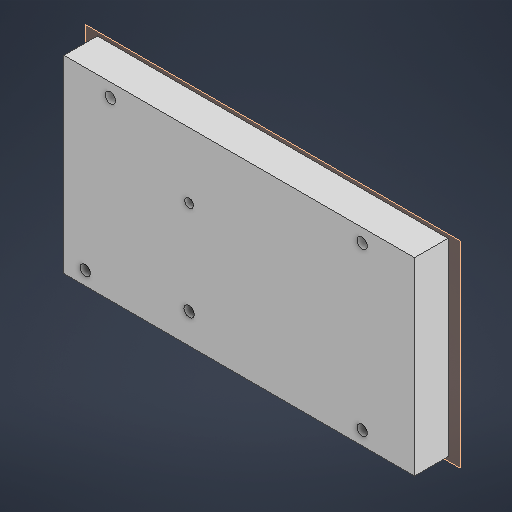
# Autodesk Inventor part: SAFRS-P-0040
Saved by Autodesk Inventor 2026.2 (Build 302298000, 298)
## iProperties
Created: 2025-11-26
Part Number: SAFRS-P-0040
Material: 일반
Document SubType Name: Modeling
Designer: jaewook
Density: 1 g/cm^3
Appearance: 기본값
Author: jaewook
Title: Mega Base
Autodesk Inventor part; units mm, degrees
ref_plane "YZ Plane" through (0, 0, 0) normal (1, 0, 0) x (0, 1, 0)
ref_plane "XZ Plane" through (0, 0, 0) normal (0, 1, 0) x (-1, 0, 0)
ref_plane "XY Plane" through (0, 0, 0) normal (0, 0, 1) x (1, 0, 0)
ref_plane "작업 평면1" through (0, 0, 0) normal (0, 0, 1) x (1, 0, 0)
sketch "스케치1" plane through (0, 0, 0) normal (0, 0, 1) x (1, 0, 0)
  line L0 (-103.1, 54.9162) -> (1.5, 54.9162)
  line L1 (1.5, 54.9162) -> (1.5, -1.5)
  line L2 (1.5, -1.5) -> (-103.1, -1.5)
  line L3 (-103.1, -1.5) -> (-103.1, 54.9162)
  line L4 (0, 1.524) -> (0, 51.8922) projected
  line L5 (-99.06, 40.7162) -> (-101.6, 38.1762) projected
  line L6 (-101.6, 38.1762) -> (-101.6, 3.556) projected
  line L7 (-101.6, 3.556) -> (-98.044, 0) projected
  line L8 (-98.044, 0) -> (-1.524, 0) projected
  line L9 (-1.524, 0) -> (0, 1.524) projected
  line L10 (0, 1.524) -> (0, 51.8922) projected
  line L11 (0, 51.8922) -> (-1.524, 53.4162) projected
  line L12 (-1.524, 53.4162) -> (-97.2966, 53.4162) projected
  line L13 (-97.2966, 53.4162) -> (-99.06, 51.6528) projected
  line L14 (-99.06, 51.6528) -> (-99.06, 40.7162) projected
  circle A0 centre (-89.2556, 50.8762) radius 1.5621 projected
  circle A1 centre (-65.7479, 35.4347) radius 1.3153 projected
  circle A2 centre (-65.7479, 7.4185) radius 1.5621 projected
  circle A3 centre (-96.7486, 2.54) radius 1.5621 projected
  circle A4 centre (-14.1224, 2.54) radius 1.5621 projected
  circle A5 centre (-14.1224, 50.8762) radius 1.5621 projected
  line L15 (-91.7703, 3.1886) -> (-92.8414, 3.1886) projected
  line L16 (-91.7703, 1.1751) -> (-91.7703, 3.1886) projected
  line L17 (-92.8414, 1.1751) -> (-91.7703, 1.1751) projected
  line L18 (-92.8414, 3.1886) -> (-92.8414, 1.1751) projected
  line L19 (-86.6903, 1.1751) -> (-86.6903, 3.1886) projected
  line L20 (-87.7614, 1.1751) -> (-86.6903, 1.1751) projected
  line L21 (-87.7614, 3.1886) -> (-87.7614, 1.1751) projected
  line L22 (-86.6903, 3.1886) -> (-87.7614, 3.1886) projected
  line L23 (-81.6103, 1.1751) -> (-81.6103, 3.1886) projected
  line L24 (-82.6814, 1.1751) -> (-81.6103, 1.1751) projected
  line L25 (-82.6814, 3.1886) -> (-82.6814, 1.1751) projected
  line L26 (-81.6103, 3.1886) -> (-82.6814, 3.1886) projected
  line L27 (-76.5303, 1.1751) -> (-76.5303, 3.1886) projected
  line L28 (-77.6014, 1.1751) -> (-76.5303, 1.1751) projected
  line L29 (-77.6014, 3.1886) -> (-77.6014, 1.1751) projected
  line L30 (-76.5303, 3.1886) -> (-77.6014, 3.1886) projected
  line L31 (-68.6825, 3.4297) -> (-69.7244, 3.4297) projected
  line L32 (-68.6825, 1.346) -> (-68.6825, 3.4297) projected
  line L33 (-69.7244, 1.346) -> (-68.6825, 1.346) projected
  line L34 (-69.7244, 3.4297) -> (-69.7244, 1.346) projected
  line L35 (-63.6025, 1.346) -> (-63.6025, 3.4297) projected
  line L36 (-64.6444, 1.346) -> (-63.6025, 1.346) projected
  line L37 (-64.6444, 3.4297) -> (-64.6444, 1.346) projected
  line L38 (-63.6025, 3.4297) -> (-64.6444, 3.4297) projected
  line L39 (-58.5225, 1.346) -> (-58.5225, 3.4297) projected
  line L40 (-59.5644, 1.346) -> (-58.5225, 1.346) projected
  line L41 (-59.5644, 3.4297) -> (-59.5644, 1.346) projected
  line L42 (-58.5225, 3.4297) -> (-59.5644, 3.4297) projected
  line L43 (-53.4425, 1.346) -> (-53.4425, 3.4297) projected
  line L44 (-54.4844, 1.346) -> (-53.4425, 1.346) projected
  line L45 (-54.4844, 3.4297) -> (-54.4844, 1.346) projected
  line L46 (-53.4425, 3.4297) -> (-54.4844, 3.4297) projected
  line L47 (-45.4737, 3.6867) -> (-46.5774, 3.6867) projected
  line L48 (-45.4737, 1.6118) -> (-45.4737, 3.6867) projected
  line L49 (-46.5774, 1.6118) -> (-45.4737, 1.6118) projected
  line L50 (-46.5774, 3.6867) -> (-46.5774, 1.6118) projected
  line L51 (-40.3937, 1.6118) -> (-40.3937, 3.6867) projected
  line L52 (-41.4974, 1.6118) -> (-40.3937, 1.6118) projected
  line L53 (-41.4974, 3.6867) -> (-41.4974, 1.6118) projected
  line L54 (-40.3937, 3.6867) -> (-41.4974, 3.6867) projected
  line L55 (-35.3137, 1.6118) -> (-35.3137, 3.6867) projected
  line L56 (-36.4174, 1.6118) -> (-35.3137, 1.6118) projected
  line L57 (-36.4174, 3.6867) -> (-36.4174, 1.6118) projected
  line L58 (-35.3137, 3.6867) -> (-36.4174, 3.6867) projected
  circle A6 centre (-97.5648, 7.2848) radius 0.5739 projected
  circle A7 centre (-95.0248, 7.2848) radius 0.5739 projected
  circle A8 centre (-95.0248, 9.8248) radius 0.5739 projected
  circle A9 centre (-95.0248, 12.3648) radius 0.5739 projected
  circle A10 centre (-95.0248, 14.9048) radius 0.5739 projected
  circle A11 centre (-95.0248, 17.4448) radius 0.5739 projected
  circle A12 centre (-95.0248, 19.9848) radius 0.5739 projected
  circle A13 centre (-95.0248, 22.5248) radius 0.5739 projected
  circle A14 centre (-95.0248, 25.0648) radius 0.5739 projected
  circle A15 centre (-95.0248, 27.6048) radius 0.5739 projected
  circle A16 centre (-95.0248, 30.1448) radius 0.5739 projected
  circle A17 centre (-95.0248, 32.6848) radius 0.5739 projected
  circle A18 centre (-95.0248, 35.2248) radius 0.5739 projected
  circle A19 centre (-95.0248, 37.7648) radius 0.5739 projected
  circle A20 centre (-95.0248, 40.3048) radius 0.5739 projected
  circle A21 centre (-95.0248, 42.8448) radius 0.5739 projected
  circle A22 centre (-95.0248, 45.3848) radius 0.5739 projected
  circle A23 centre (-95.0248, 47.9248) radius 0.5739 projected
  circle A24 centre (-95.0248, 50.4648) radius 0.5739 projected
  line L59 (-81.8933, 50.0717) -> (-81.8933, 51.6679) projected
  line L60 (-82.3984, 50.0717) -> (-81.8933, 50.0717) projected
  line L61 (-82.3984, 51.6679) -> (-82.3984, 50.0717) projected
  line L62 (-81.8933, 51.6679) -> (-82.3984, 51.6679) projected
  line L63 (-76.8133, 50.0717) -> (-76.8133, 51.6679) projected
  line L64 (-77.3184, 50.0717) -> (-76.8133, 50.0717) projected
  line L65 (-77.3184, 51.6679) -> (-77.3184, 50.0717) projected
  line L66 (-76.8133, 51.6679) -> (-77.3184, 51.6679) projected
  line L67 (-71.7333, 50.0717) -> (-71.7333, 51.6679) projected
  line L68 (-72.2384, 50.0717) -> (-71.7333, 50.0717) projected
  line L69 (-72.2384, 51.6679) -> (-72.2384, 50.0717) projected
  line L70 (-71.7333, 51.6679) -> (-72.2384, 51.6679) projected
  line L71 (-63.4227, 51.9137) -> (-64.2563, 51.9137) projected
  line L72 (-63.4227, 50.0717) -> (-63.4227, 51.9137) projected
  line L73 (-64.2563, 50.0717) -> (-63.4227, 50.0717) projected
  line L74 (-64.2563, 51.9137) -> (-64.2563, 50.0717) projected
  line L75 (-58.3427, 50.0717) -> (-58.3427, 51.9137) projected
  line L76 (-59.1763, 50.0717) -> (-58.3427, 50.0717) projected
  line L77 (-59.1763, 51.9137) -> (-59.1763, 50.0717) projected
  line L78 (-58.3427, 51.9137) -> (-59.1763, 51.9137) projected
  line L79 (-53.2627, 50.0717) -> (-53.2627, 51.9137) projected
  line L80 (-54.0963, 50.0717) -> (-53.2627, 50.0717) projected
  line L81 (-54.0963, 51.9137) -> (-54.0963, 50.0717) projected
  line L82 (-53.2627, 51.9137) -> (-54.0963, 51.9137) projected
  line L83 (-48.1827, 50.0717) -> (-48.1827, 51.9137) projected
  line L84 (-49.0163, 50.0717) -> (-48.1827, 50.0717) projected
  line L85 (-49.0163, 51.9137) -> (-49.0163, 50.0717) projected
  line L86 (-48.1827, 51.9137) -> (-49.0163, 51.9137) projected
  line L87 (-41.4974, 51.9137) -> (-42.4723, 51.9137) projected
  line L88 (-41.4974, 50.0717) -> (-41.4974, 51.9137) projected
  line L89 (-42.4723, 50.0717) -> (-41.4974, 50.0717) projected
  line L90 (-42.4723, 51.9137) -> (-42.4723, 50.0717) projected
  line L91 (-36.4174, 50.0717) -> (-36.4174, 51.9137) projected
  line L92 (-37.3923, 50.0717) -> (-36.4174, 50.0717) projected
  line L93 (-37.3923, 51.9137) -> (-37.3923, 50.0717) projected
  line L94 (-36.4174, 51.9137) -> (-37.3923, 51.9137) projected
  line L95 (-31.3374, 50.0717) -> (-31.3374, 51.9137) projected
  line L96 (-32.3123, 50.0717) -> (-31.3374, 50.0717) projected
  line L97 (-32.3123, 51.9137) -> (-32.3123, 50.0717) projected
  line L98 (-31.3374, 51.9137) -> (-32.3123, 51.9137) projected
  line L99 (-26.2574, 50.0717) -> (-26.2574, 51.9137) projected
  line L100 (-27.2323, 50.0717) -> (-26.2574, 50.0717) projected
  line L101 (-27.2323, 51.9137) -> (-27.2323, 50.0717) projected
  line L102 (-26.2574, 51.9137) -> (-27.2323, 51.9137) projected
  circle A25 centre (-20.5945, 47.6784) radius 0.5437 projected
  circle A26 centre (-18.0545, 47.6784) radius 0.5437 projected
  circle A27 centre (-20.5945, 45.1384) radius 0.5437 projected
  circle A28 centre (-15.5145, 45.1384) radius 0.5437 projected
  circle A29 centre (-5.7466, 39.5769) radius 0.4144 projected
  circle A30 centre (-5.7466, 37.0369) radius 0.4144 projected
  line L103 (-7.393, 4.043) -> (-10.0091, 4.043) projected
  line L104 (-7.393, 3.3305) -> (-7.393, 4.043) projected
  line L105 (-10.0091, 3.3305) -> (-7.393, 3.3305) projected
  line L106 (-10.0091, 4.043) -> (-10.0091, 3.3305) projected
  line L107 (-2.4767, 32.5537) -> (-4.2776, 32.5537) projected
  line L108 (-2.4767, 31.6979) -> (-2.4767, 32.5537) projected
  line L109 (-4.2776, 31.6979) -> (-2.4767, 31.6979) projected
  line L110 (-4.2776, 32.5537) -> (-4.2776, 31.6979) projected
  line L111 (-2.249, 44.6927) -> (-4.5054, 44.6927) projected
  line L112 (-2.249, 43.8153) -> (-2.249, 44.6927) projected
  line L113 (-4.5054, 43.8153) -> (-2.249, 43.8153) projected
  line L114 (-4.5054, 44.6927) -> (-4.5054, 43.8153) projected
  line L115 (-5.2737, 10.2292) -> (-5.7128, 10.2292) projected
  line L116 (-5.2737, 7.3652) -> (-5.2737, 10.2292) projected
  line L117 (-5.7128, 7.3652) -> (-5.2737, 7.3652) projected
  line L118 (-5.7128, 10.2292) -> (-5.7128, 7.3652) projected
  circle A31 centre (-8.2866, 37.0369) radius 0.4144 projected
  line L119 (-11.4599, 10.2292) -> (-12.1472, 10.2292) projected
  line L120 (-11.4599, 7.3652) -> (-11.4599, 10.2292) projected
  line L121 (-12.1472, 7.3652) -> (-11.4599, 7.3652) projected
  line L122 (-12.1472, 10.2292) -> (-12.1472, 7.3652) projected
  circle A32 centre (-18.0545, 45.1384) radius 0.5437 projected
  circle A33 centre (-15.5145, 47.6784) radius 0.5437 projected
  circle A34 centre (-8.2866, 39.5769) radius 0.4144 projected
  line L123 (-23.7174, 50.0717) -> (-23.7174, 51.9137) projected
  line L124 (-24.6923, 50.0717) -> (-23.7174, 50.0717) projected
  line L125 (-24.6923, 51.9137) -> (-24.6923, 50.0717) projected
  line L126 (-23.7174, 51.9137) -> (-24.6923, 51.9137) projected
  line L127 (-28.7974, 50.0717) -> (-28.7974, 51.9137) projected
  line L128 (-29.7723, 50.0717) -> (-28.7974, 50.0717) projected
  line L129 (-29.7723, 51.9137) -> (-29.7723, 50.0717) projected
  line L130 (-28.7974, 51.9137) -> (-29.7723, 51.9137) projected
  line L131 (-33.8774, 50.0717) -> (-33.8774, 51.9137) projected
  line L132 (-34.8523, 50.0717) -> (-33.8774, 50.0717) projected
  line L133 (-34.8523, 51.9137) -> (-34.8523, 50.0717) projected
  line L134 (-33.8774, 51.9137) -> (-34.8523, 51.9137) projected
  line L135 (-38.9574, 50.0717) -> (-38.9574, 51.9137) projected
  line L136 (-39.9323, 50.0717) -> (-38.9574, 50.0717) projected
  line L137 (-39.9323, 51.9137) -> (-39.9323, 50.0717) projected
  line L138 (-38.9574, 51.9137) -> (-39.9323, 51.9137) projected
  line L139 (-45.6427, 50.0717) -> (-45.6427, 51.9137) projected
  line L140 (-46.4763, 50.0717) -> (-45.6427, 50.0717) projected
  line L141 (-46.4763, 51.9137) -> (-46.4763, 50.0717) projected
  line L142 (-45.6427, 51.9137) -> (-46.4763, 51.9137) projected
  line L143 (-50.7227, 50.0717) -> (-50.7227, 51.9137) projected
  line L144 (-51.5563, 50.0717) -> (-50.7227, 50.0717) projected
  line L145 (-51.5563, 51.9137) -> (-51.5563, 50.0717) projected
  line L146 (-50.7227, 51.9137) -> (-51.5563, 51.9137) projected
  line L147 (-55.8027, 50.0717) -> (-55.8027, 51.9137) projected
  line L148 (-56.6363, 50.0717) -> (-55.8027, 50.0717) projected
  line L149 (-56.6363, 51.9137) -> (-56.6363, 50.0717) projected
  line L150 (-55.8027, 51.9137) -> (-56.6363, 51.9137) projected
  line L151 (-60.8827, 50.0717) -> (-60.8827, 51.9137) projected
  line L152 (-61.7163, 50.0717) -> (-60.8827, 50.0717) projected
  line L153 (-61.7163, 51.9137) -> (-61.7163, 50.0717) projected
  line L154 (-60.8827, 51.9137) -> (-61.7163, 51.9137) projected
  line L155 (-69.1933, 50.0717) -> (-69.1933, 51.6679) projected
  line L156 (-69.6984, 50.0717) -> (-69.1933, 50.0717) projected
  line L157 (-69.6984, 51.6679) -> (-69.6984, 50.0717) projected
  line L158 (-69.1933, 51.6679) -> (-69.6984, 51.6679) projected
  line L159 (-74.2733, 50.0717) -> (-74.2733, 51.6679) projected
  line L160 (-74.7784, 50.0717) -> (-74.2733, 50.0717) projected
  line L161 (-74.7784, 51.6679) -> (-74.7784, 50.0717) projected
  line L162 (-74.2733, 51.6679) -> (-74.7784, 51.6679) projected
  line L163 (-79.3533, 50.0717) -> (-79.3533, 51.6679) projected
  line L164 (-79.8584, 50.0717) -> (-79.3533, 50.0717) projected
  line L165 (-79.8584, 51.6679) -> (-79.8584, 50.0717) projected
  line L166 (-79.3533, 51.6679) -> (-79.8584, 51.6679) projected
  line L167 (-84.4333, 50.0717) -> (-84.4333, 51.6679) projected
  line L168 (-84.9384, 50.0717) -> (-84.4333, 50.0717) projected
  line L169 (-84.9384, 51.6679) -> (-84.9384, 50.0717) projected
  line L170 (-84.4333, 51.6679) -> (-84.9384, 51.6679) projected
  circle A35 centre (-97.5648, 50.4648) radius 0.5739 projected
  circle A36 centre (-97.5648, 47.9248) radius 0.5739 projected
  circle A37 centre (-97.5648, 45.3848) radius 0.5739 projected
  circle A38 centre (-97.5648, 42.8448) radius 0.5739 projected
  circle A39 centre (-97.5648, 40.3048) radius 0.5739 projected
  circle A40 centre (-97.5648, 37.7648) radius 0.5739 projected
  circle A41 centre (-97.5648, 35.2248) radius 0.5739 projected
  circle A42 centre (-97.5648, 32.6848) radius 0.5739 projected
  circle A43 centre (-97.5648, 30.1448) radius 0.5739 projected
  circle A44 centre (-97.5648, 27.6048) radius 0.5739 projected
  circle A45 centre (-97.5648, 25.0648) radius 0.5739 projected
  circle A46 centre (-97.5648, 22.5248) radius 0.5739 projected
  circle A47 centre (-97.5648, 19.9848) radius 0.5739 projected
  circle A48 centre (-97.5648, 17.4448) radius 0.5739 projected
  circle A49 centre (-97.5648, 14.9048) radius 0.5739 projected
  circle A50 centre (-97.5648, 12.3648) radius 0.5739 projected
  circle A51 centre (-97.5648, 9.8248) radius 0.5739 projected
  line L171 (-86.9733, 51.6679) -> (-87.4784, 51.6679) projected
  line L172 (-86.9733, 50.0717) -> (-86.9733, 51.6679) projected
  line L173 (-87.4784, 50.0717) -> (-86.9733, 50.0717) projected
  line L174 (-87.4784, 51.6679) -> (-87.4784, 50.0717) projected
  line L175 (-32.7737, 1.6118) -> (-32.7737, 3.6867) projected
  line L176 (-33.8774, 1.6118) -> (-32.7737, 1.6118) projected
  line L177 (-33.8774, 3.6867) -> (-33.8774, 1.6118) projected
  line L178 (-32.7737, 3.6867) -> (-33.8774, 3.6867) projected
  line L179 (-37.8537, 1.6118) -> (-37.8537, 3.6867) projected
  line L180 (-38.9574, 1.6118) -> (-37.8537, 1.6118) projected
  line L181 (-38.9574, 3.6867) -> (-38.9574, 1.6118) projected
  line L182 (-37.8537, 3.6867) -> (-38.9574, 3.6867) projected
  line L183 (-42.9337, 1.6118) -> (-42.9337, 3.6867) projected
  line L184 (-44.0374, 1.6118) -> (-42.9337, 1.6118) projected
  line L185 (-44.0374, 3.6867) -> (-44.0374, 1.6118) projected
  line L186 (-42.9337, 3.6867) -> (-44.0374, 3.6867) projected
  line L187 (-50.9025, 1.346) -> (-50.9025, 3.4297) projected
  line L188 (-51.9444, 1.346) -> (-50.9025, 1.346) projected
  line L189 (-51.9444, 3.4297) -> (-51.9444, 1.346) projected
  line L190 (-50.9025, 3.4297) -> (-51.9444, 3.4297) projected
  line L191 (-55.9825, 1.346) -> (-55.9825, 3.4297) projected
  line L192 (-57.0244, 1.346) -> (-55.9825, 1.346) projected
  line L193 (-57.0244, 3.4297) -> (-57.0244, 1.346) projected
  line L194 (-55.9825, 3.4297) -> (-57.0244, 3.4297) projected
  line L195 (-61.0625, 1.346) -> (-61.0625, 3.4297) projected
  line L196 (-62.1044, 1.346) -> (-61.0625, 1.346) projected
  line L197 (-62.1044, 3.4297) -> (-62.1044, 1.346) projected
  line L198 (-61.0625, 3.4297) -> (-62.1044, 3.4297) projected
  line L199 (-66.1425, 1.346) -> (-66.1425, 3.4297) projected
  line L200 (-67.1844, 1.346) -> (-66.1425, 1.346) projected
  line L201 (-67.1844, 3.4297) -> (-67.1844, 1.346) projected
  line L202 (-66.1425, 3.4297) -> (-67.1844, 3.4297) projected
  line L203 (-73.9903, 1.1751) -> (-73.9903, 3.1886) projected
  line L204 (-75.0614, 1.1751) -> (-73.9903, 1.1751) projected
  line L205 (-75.0614, 3.1886) -> (-75.0614, 1.1751) projected
  line L206 (-73.9903, 3.1886) -> (-75.0614, 3.1886) projected
  line L207 (-79.0703, 1.1751) -> (-79.0703, 3.1886) projected
  line L208 (-80.1414, 1.1751) -> (-79.0703, 1.1751) projected
  line L209 (-80.1414, 3.1886) -> (-80.1414, 1.1751) projected
  line L210 (-79.0703, 3.1886) -> (-80.1414, 3.1886) projected
  line L211 (-84.1503, 1.1751) -> (-84.1503, 3.1886) projected
  line L212 (-85.2214, 1.1751) -> (-84.1503, 1.1751) projected
  line L213 (-85.2214, 3.1886) -> (-85.2214, 1.1751) projected
  line L214 (-84.1503, 3.1886) -> (-85.2214, 3.1886) projected
  line L215 (-89.2303, 1.1751) -> (-89.2303, 3.1886) projected
  line L216 (-90.3014, 1.1751) -> (-89.2303, 1.1751) projected
  line L217 (-90.3014, 3.1886) -> (-90.3014, 1.1751) projected
  line L218 (-89.2303, 3.1886) -> (-90.3014, 3.1886) projected
  point P0 (0, 0)
  dimension "d0" = 1.5
  dimension "d1" = 1.5
  dimension "d2" = 1.5
  dimension "d3" = 1.5
  constraints: 8 end point, 2 parallel, 1 horizontal, 1 perpendicular
  measures "d0" distance between parallel lines of L12 L0
  measures "d1" distance between parallel lines of L6 L3
  measures "d2" distance between parallel lines of L2 L8
  measures "d3" distance between parallel lines of L4 L1
extrude "돌출1" add sketch "스케치1" along normal blind 10 contours L0 L1 L2 L3 | L9 L8 L7 L6 L5 L14 L13 L12 L11 L4 | L16 L17 L18 L15 | L20 L21 L22 L19 | L24 L25 L26 L23 | L28 L29 L30 L27 | L32 L33 L34 L31 | L36 L37 L38 L35 | L40 L41 L42 L39 | L44 L45 L46 L43 | L48 L49 L50 L47 | L52 L53 L54 L51 | L56 L57 L58 L55 | A6 | A7 | A8 | A9 | A10 | A11 | A12 | A13 | A14 | A15 | A16 | A17 | A18 | A19 | A20 | A21 | A22 | A23 | A24 | L60 L61 L62 L59 | L64 L65 L66 L63 | L68 L69 L70 L67 | L72 L73 L74 L71 | L76 L77 L78 L75 | L80 L81 L82 L79 | L84 L85 L86 L83 | L88 L89 L90 L87 | L92 L93 L94 L91 | L96 L97 L98 L95 | L100 L101 L102 L99 | A25 | A26 | A27 | A28 | A29 | A30 | L104 L105 L106 L103 | L108 L109 L110 L107 | L112 L113 L114 L111 | L116 L117 L118 L115 | A31 | L120 L121 L122 L119 | A32 | A33 | A34 | L124 L125 L126 L123 | L128 L129 L130 L127 | L132 L133 L134 L131 | L136 L137 L138 L135 | L140 L141 L142 L139 | L144 L145 L146 L143 | L148 L149 L150 L147 | L152 L153 L154 L151 | L156 L157 L158 L155 | L160 L161 L162 L159 | L164 L165 L166 L163 | L168 L169 L170 L167 | A35 | A36 | A37 | A38 | A39 | A40 | A41 | A42 | A43 | A44 | A45 | A46 | A47 | A48 | A49 | A50 | A51 | L172 L173 L174 L171 | L176 L177 L178 L175 | L180 L181 L182 L179 | L184 L185 L186 L183 | L188 L189 L190 L187 | L192 L193 L194 L191 | L196 L197 L198 L195 | L200 L201 L202 L199 | L204 L205 L206 L203 | L208 L209 L210 L207 | L212 L213 L214 L211 | L216 L217 L218 L215
